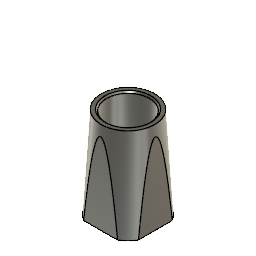
GPU jack base v2 (Autodesk Fusion 360 design; units mm, degrees)
Autodesk Fusion 360 part; units mm, degrees
sketch "Sketch1" plane through (0, 0, 0) normal (0, 1, 0) x (1, 0, 0)
  line L0 (-9, 0) -> (9, 0)
  line L1 (9, 0) -> (9, -30)
  line L2 (9, -30) -> (-9, -30)
  line L3 (-9, -30) -> (-9, 0)
  dimension "d1" = 18
  dimension "d2" = 30
  constraint horizontal L0
  constraint vertical L1
  constraint horizontal L2
  constraint vertical L3
  measures "d1" distance of L0.start L0.end
  measures "d2" distance of L0.start L2.end
extrude "Extrude1" add sketch "Sketch1" along normal blind 18
sketch "Sketch3" plane through (0, 0, 30) normal (0, 0, 1) x (-1, 0, 0)
  line L0 (9, 0) -> (-9, 0)
  line L1 (-9, 0) -> (-9, -18)
  line L2 (-9, -18) -> (9, -18)
  line L3 (9, -18) -> (9, 0)
  circle A0 centre (0, -9) radius 7.05
  dimension "d6" = 14.1
  measures "d6" diameter of A0
extrude "Extrude2" cut sketch "Sketch3" against normal blind 12 contours A0
chamfer "Chamfer1" distance 0.5 angle 45 1 edges at (6.5729, 6.4506, 30)
move_body "Move1" bodies 1 to x (1, 0, 0) y (0, 1, 0) z (0, 0, 1) at (0, -9, 0)
sketch "Sketch4" plane through (0, 0, 0) normal (0, 1, 0) x (1, 0, 0)
  line L0 (6, -77) -> (11, 7)
  line L1 (11, 7) -> (65, -11)
  line L2 (65, -11) -> (6, -77)
revolve "Revolve1" cut sketch "Sketch4" angle 360 about axis through (0, 0, 1.75) along (0, 0, 1)
equation "d2 = 18 mm + 12 mm"
